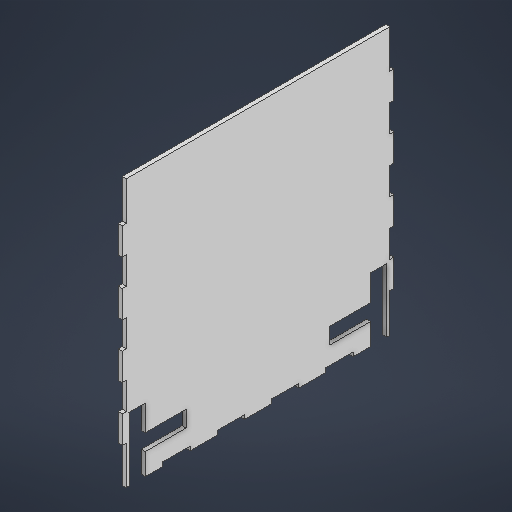
# Autodesk Inventor part: outsidewall_left
Saved by Autodesk Inventor 2026.2 (Build 302298000, 298)
## iProperties
Created: 2026-02-16
Part Number: outsidewall_left
Material: Generic
Document SubType Name: Modeling
Designer: ruhir
Density: 1 g/cm^3
Appearance: Default
Author: ruhir
Autodesk Inventor part; units mm, degrees
ref_plane "YZ Plane" through (0, 0, 0) normal (1, 0, 0) x (0, 1, 0)
ref_plane "XZ Plane" through (0, 0, 0) normal (0, 1, 0) x (-1, 0, 0)
ref_plane "XY Plane" through (0, 0, 0) normal (0, 0, 1) x (1, 0, 0)
sketch "Sketch1" plane through (0, 0, 0) normal (1, 0, 0) x (0, 1, 0)
  line L0 (3, 191.4188) -> (-194, 191.4188) construction
  line L1 (-194, 191.4188) -> (-194, -8.5812) construction
  line L2 (-194, -8.5812) -> (3, -8.5812) construction
  line L3 (3, -8.5812) -> (3, 191.4188) construction
  line L4 (0, 188.4188) -> (-191, 188.4188) construction
  line L5 (-191, 188.4188) -> (-191, -5.5812) construction
  line L6 (-191, -5.5812) -> (0, -5.5812) construction
  line L7 (0, -5.5812) -> (0, 188.4188) construction
  line L8 (-165.5, -5.5812) -> (-165.5, -8.5812) construction
  line L9 (-194, -5.5812) -> (-165.5, -5.5812)
  line L10 (-165.5, -5.5812) -> (-165.5, -8.5812)
  line L11 (-165.5, -8.5812) -> (-145.5, -8.5812)
  line L12 (-145.5, -8.5812) -> (-145.5, -5.5812)
  line L13 (-145.5, -5.5812) -> (-125.5, -5.5812)
  line L14 (-125.5, -5.5812) -> (-125.5, -8.5812)
  line L15 (3, -5.5812) -> (-25.5, -5.5812)
  line L16 (-25.5, -5.5812) -> (-25.5, -8.5812)
  line L17 (-25.5, -8.5812) -> (-45.5, -8.5812)
  line L18 (-45.5, -8.5812) -> (-45.5, -5.5812)
  line L19 (-45.5, -5.5812) -> (-65.5, -5.5812)
  line L20 (-65.5, -5.5812) -> (-65.5, -8.5812)
  line L21 (-65.5, -8.5812) -> (-85.5, -8.5812)
  line L22 (-85.5, -8.5812) -> (-85.5, -5.5812)
  line L23 (-85.5, -5.5812) -> (-105.5, -5.5812)
  line L24 (-105.5, -5.5812) -> (-105.5, -8.5812)
  line L25 (-105.5, -8.5812) -> (-125.5, -8.5812)
  line L26 (-194, 188.4188) -> (-165.5, 188.4188)
  line L27 (-165.5, 188.4188) -> (-165.5, 191.4188)
  line L28 (3, 188.4188) -> (-25.5, 188.4188)
  line L29 (-25.5, 188.4188) -> (-25.5, 191.4188)
  line L30 (-25.5, 191.4188) -> (-45.5, 191.4188)
  line L31 (-45.5, 191.4188) -> (-45.5, 188.4188)
  line L32 (-45.5, 188.4188) -> (-65.5, 188.4188)
  line L33 (-65.5, 188.4188) -> (-65.5, 191.4188)
  line L34 (-65.5, 191.4188) -> (-85.5, 191.4188)
  line L35 (-85.5, 191.4188) -> (-85.5, 188.4188)
  line L36 (-85.5, 188.4188) -> (-105.5, 188.4188)
  line L37 (-105.5, 188.4188) -> (-105.5, 191.4188)
  line L38 (-105.5, 191.4188) -> (-125.5, 191.4188)
  line L39 (-125.5, 191.4188) -> (-125.5, 188.4188)
  line L40 (-125.5, 188.4188) -> (-145.5, 188.4188)
  line L41 (-145.5, 188.4188) -> (-145.5, 191.4188)
  line L42 (-145.5, 191.4188) -> (-165.5, 191.4188)
  line L43 (-194, 188.4188) -> (-194, 161.4188)
  line L44 (-194, 161.4188) -> (-191, 161.4188)
  line L45 (-191, 161.4188) -> (-191, 141.4188)
  line L46 (-191, 141.4188) -> (-194, 141.4188)
  line L47 (-194, 141.4188) -> (-194, 121.4188)
  line L48 (-194, 121.4188) -> (-191, 121.4188)
  line L49 (-194, -5.5812) -> (-194, 21.4188)
  line L50 (-194, 21.4188) -> (-191, 21.4188)
  line L51 (-191, 21.4188) -> (-191, 41.4188)
  line L52 (-191, 41.4188) -> (-194, 41.4188)
  line L53 (-194, 41.4188) -> (-194, 61.4188)
  line L54 (-194, 61.4188) -> (-191, 61.4188)
  line L55 (-191, 61.4188) -> (-191, 81.4188)
  line L56 (-191, 81.4188) -> (-194, 81.4188)
  line L57 (-194, 81.4188) -> (-194, 101.4188)
  line L58 (-194, 101.4188) -> (-191, 101.4188)
  line L59 (-191, 101.4188) -> (-191, 121.4188)
  line L60 (3, -5.5812) -> (3, 188.4188)
  line L61 (-194, 186.4008) -> (-146.985, 186.4008)
  line L62 (-146.985, 186.4008) -> (-146.985, 174.4008)
  line L63 (-177.985, 174.4008) -> (-177.985, 144.4008)
  line L64 (-177.985, 144.4008) -> (-165.985, 144.4008)
  line L65 (-165.985, 144.4008) -> (-165.985, 174.4008)
  line L66 (-194, -3.5632) -> (-146.985, -3.5632)
  line L67 (-146.985, -3.5632) -> (-146.985, 8.4368)
  line L68 (-146.985, 8.4368) -> (-165.985, 8.4368)
  line L69 (-165.985, 8.4368) -> (-165.985, 38.4368)
  line L70 (-165.985, 38.4368) -> (-177.985, 38.4368)
  line L71 (-177.985, 38.4368) -> (-177.985, 8.4368)
  line L72 (-177.985, 8.4368) -> (-194, 8.4368)
  line L73 (-177.985, 174.4008) -> (-194, 174.4008)
  line L74 (-146.985, 174.4008) -> (-165.985, 174.4008)
  point P0 (0, 0)
  point P1 (-170.4925, 186.4008)
  point P2 (-194, 174.9188)
  dimension "d0" = 197
  dimension "d1" = 200
  dimension "d2" = 3
  dimension "d3" = 3
  dimension "d4" = 3
  dimension "d5" = 3
  dimension "d6" = 3
  dimension "d7" = 3
  dimension "d8" = 3
  dimension "d9" = 3
  dimension "d11" = 28.5
  dimension "d12" = 20
  dimension "d13" = 20
  dimension "d14" = 28.5
  dimension "d15" = 20
  dimension "d16" = 20
  dimension "d17" = 20
  dimension "d18" = 20
  dimension "d19" = 28.5
  dimension "d20" = 28.5
  dimension "d21" = 20
  dimension "d22" = 20
  dimension "d23" = 20
  dimension "d24" = 20
  dimension "d25" = 20
  dimension "d26" = 20
  dimension "d27" = 27
  dimension "d28" = 20
  dimension "d29" = 20
  dimension "d30" = 27
  dimension "d31" = 20
  dimension "d32" = 20
  dimension "d33" = 20
  dimension "d34" = 20
  dimension "d35" = 5.018
  dimension "d37" = 47.015
  dimension "d38" = 12
  dimension "d39" = 19
  dimension "d40" = 30
  dimension "d41" = 12
  dimension "d42" = 16.015
  dimension "d43" = 5.018
  dimension "d47" = 47.015
  dimension "d48" = 30
  dimension "d49" = 12
  dimension "d50" = 12
  dimension "d51" = 19
  dimension "d52" = 16.015
  constraints: 138 end point, 20 vertical, 14 horizontal, 10 perpendicular, 8 point on line, 2 midpoint, 68 other
  measures "d0" distance of L3.start point (-194, -8.581)
  measures "d1" distance of point (-194, 191.419) point (-194, -8.581)
  measures "d3" distance from line of L3 L7.start
  measures "d9" distance from line of L3 L7.end
  measures "d11" distance of L9.start L8.start
  measures "d12" distance of L8.end L11.end
  measures "d13" distance of L12.end L13.end
  measures "d14" distance of L15.start L15.end
  measures "d15" distance of L16.end L17.end
  measures "d16" distance of L18.end L19.end
  measures "d17" distance of L20.end L21.end
  measures "d18" distance of L22.end L23.end
  measures "d19" distance of L26.start L26.end
  measures "d20" distance of L28.start L28.end
  measures "d21" distance of L29.end L30.end
  measures "d22" distance of L31.end L32.end
  measures "d23" distance of L33.end L34.end
  measures "d24" distance of L35.end L36.end
  measures "d25" distance of L37.end L38.end
  measures "d26" distance of L39.end L40.end
  measures "d27" distance of L26.start L43.end
  measures "d28" distance of L44.end L45.end
  measures "d29" distance of L46.end L47.end
  measures "d30" distance of L9.start L49.end
  measures "d31" distance of L50.end L51.end
  measures "d32" distance of L52.end L53.end
  measures "d33" distance of L54.end L55.end
  measures "d34" distance of L56.end L57.end
  measures "d37" distance of L66.end L66.start
  measures "d38" distance of L66.end L67.end
  measures "d39" distance of L68.end L67.end
  measures "d40" distance of L69.end L68.end
  measures "d41" distance of L70.end L69.end
  measures "d42" distance of L72.end L71.end
  measures "d47" distance of L61.start L61.end
  measures "d48" distance of L63.end L63.start
  measures "d49" distance of L63.end L64.end
  measures "d50" distance of L62.end L61.end
  measures "d51" distance of L62.end L65.end
  measures "d52" horizontal distance of point (-194, 174.919) L63.start
extrude "Extrusion1" add sketch "Sketch1" along normal blind 3 contours L49 L66 L67 L68 L69 L70 L71 L72 L50 L51 L52 L53 L54 L55 L56 L57 L58 L59 L48 L47 L46 L45 L44 L43 L73 L63 L64 L65 L74 L62 L61 L26 L27 L42 L41 L40 L39 L38 L37 L36 L35 L34 L33 L32 L31 L30 L29 L28 L60 L15 L16 L17 L18 L19 L20 L21 L22 L23 L24 L25 L14 L13 L12 L11 L10 L9
body "Solid1"
